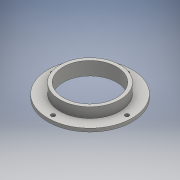
# Autodesk Inventor part: AcoplecN°2
Saved by Autodesk Inventor 2016 (Build 200138000, 138)
## iProperties
Created: 2017-08-31
Part Number: AcoplecN°2
Material: Genérico
Document SubType Name: Modeling
Designer: Alumno
Density: 1 g/cm^3
Appearance: Valor por defecto
Author: Alumno
Autodesk Inventor part; units mm, degrees
ref_plane "YZ Plane" through (0, 0, 0) normal (1, 0, 0) x (0, 1, 0)
ref_plane "XZ Plane" through (0, 0, 0) normal (0, 1, 0) x (-1, 0, 0)
ref_plane "XY Plane" through (0, 0, 0) normal (0, 0, 1) x (1, 0, 0)
sketch "Boceto1" plane through (0, 0, 0) normal (0, 0, 1) x (1, 0, 0)
  circle A0 centre (0, 0) radius 23.85
  circle A1 centre (0, 0) radius 26.85
  dimension "d0" = 47.7
  dimension "d1" = 3
  constraints: 2 centre point, 1 coincident
  measures "d0" diameter of A0
  measures "d1" radial gap between concentric circles of A0 A1
extrude "Extrusión1" add sketch "Boceto1" along normal blind 9
sketch "Boceto2" plane through (0, 0, 0) normal (0, 0, -1) x (-1, 0, 0)
  circle A0 centre (0, 0) radius 37.5
  circle A1 centre (0, 0) radius 23.85 projected
  dimension "d4" = 75
  constraints: 1 centre point, 1 coincident
  measures "d4" diameter of A0
extrude "Extrusión2" add sketch "Boceto2" along normal blind 3
sketch "Boceto6" plane through (0, 0, 0) normal (0, 0, 1) x (1, 0, 0)
  circle A0 centre (0, 33) radius 1.8
  point P0 (0, 0)
  dimension "d19" = 3.6
  dimension "d20" = 33
  constraints: 1 centre point
  measures "d19" diameter of A0
  measures "d20" distance of point (0, 0) A0.centre
extrude "Extrusión5" cut sketch "Boceto6" against normal blind 10
pattern_circular "Patrón circular1" count 4 over 360 about axis through (0, 0, -10) along (0, 0, 1) of "Extrusión5"
